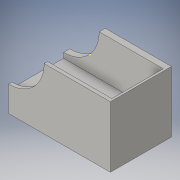
# Autodesk Inventor part: ScoopBucket
Saved by Autodesk Inventor 2016 (Build 200138000, 138)
## iProperties
Created: 2016-04-05
Part Number: ScoopBucket
Material: Generic
Document SubType Name: Modeling
Designer: Bailey
Density: 1 g/cm^3
Appearance: Default
Author: Bailey
Autodesk Inventor part; units mm, degrees
ref_plane "YZ Plane" through (0, 0, 0) normal (1, 0, 0) x (0, 1, 0)
ref_plane "XZ Plane" through (0, 0, 0) normal (0, 1, 0) x (-1, 0, 0)
ref_plane "XY Plane" through (0, 0, 0) normal (0, 0, 1) x (1, 0, 0)
sketch "Sketch1" plane through (0, 0, 0) normal (1, 0, 0) x (0, 1, 0)
  point P0 (0, 0)
sketch "Sketch2" plane through (0, 0, 0) normal (0, 1, 0) x (-1, 0, 0)
  line L0 (-6.35, 3.81) -> (6.35, 3.81)
  line L1 (6.35, 3.81) -> (6.35, -3.81)
  line L2 (6.35, -3.81) -> (-6.35, -3.81)
  line L3 (-6.35, -3.81) -> (-6.35, 3.81)
  line L4 (-6.35, 3.81) -> (6.35, -3.81) construction
  line L5 (6.35, 3.81) -> (-6.35, -3.81) construction
  point P0 (0, 0)
  dimension "d0" = 12.7
  dimension "d1" = 7.62
  constraints: 12 end point, 2 midpoint, 2 parallel, 1 horizontal, 1 perpendicular
  measures "d0" distance of L1.end L2.end
  measures "d1" distance of L0.end L1.end
extrude "Extrusion1" add sketch "Sketch2" along normal blind 7.62
sketch "Sketch3" plane through (0, 7.62, 0) normal (0, 1, 0) x (1, 0, 0)
  point P0 (0, 0)
sketch "Sketch4" plane through (-6.35, 0, 3.81) normal (0, 0, 1) x (1, 0, 0)
  line L0 (0, 7.62) -> (12.7, 7.62) projected
  circle A0 centre (0, 7.62) radius 4.445
  point P0 (6.35, 0)
  dimension "d5" = 8.89
  constraints: 1 centre point
  measures "d5" diameter of A0
extrude "Extrusion2" cut sketch "Sketch4" against normal blind 12.7
sketch "Sketch5" plane through (0, 7.62, 0) normal (0, 1, 0) x (1, 0, 0)
  point P0 (0, 0)
sketch "Sketch6" plane through (0, 7.62, 0) normal (0, 1, 0) x (1, 0, 0)
  line L0 (6.096, -3.3777) -> (-6.604, -3.3777)
  line L1 (-6.604, -3.3777) -> (-6.604, 3.0508)
  line L2 (-6.604, 3.0508) -> (6.096, 3.0508)
  line L3 (6.096, 3.0508) -> (6.096, -3.3777)
  line L4 (6.35, -3.81) -> (6.35, 3.81) projected
  point P0 (0, 0)
  dimension "d10" = 12.7
  dimension "d11" = 0.254
  constraints: 8 end point, 2 parallel, 1 horizontal, 1 perpendicular
  measures "d10" distance of L0.start L0.end
  measures "d11" distance between parallel lines of L3 L4
extrude "Extrusion3" cut sketch "Sketch6" against normal blind 5.08
body "Solid1"
